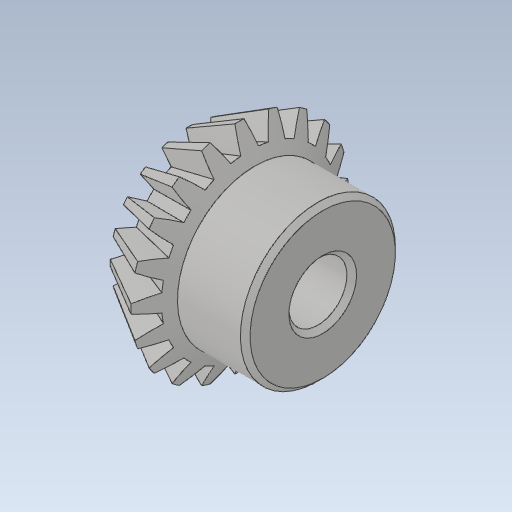
# Autodesk Inventor part: PB1-2040_On
Saved by Autodesk Inventor 2024 (Build 280153000, 153)
## iProperties
Created: 2023-09-03
Part Number: PB1-2040_On
Material: Generic
Catalog Web Link: www.cadenas.de
Description: Plastic Bevel Gears (PB)-L-
Vendor: KHK
Document SubType Name: Modeling
Designer: psAdmin
Manufacturer: KHK
Mass: 2.44535 g
Surface Area: 17.1711 cm^2
Volume: 2.44535 cm^3
Density: 1 g/cm^3
Appearance: PSOLRGB-175-175-175
Category: PARTsolutions
Company: KHK
PSOL_IDENT_0: {$CADENAS_DATA/23d-libs/khk/bevel_gears/pb_l.prj},185 {VTYP=3D},{NB=PB1-2040_On},{LINA=PB1-2040},{NN=
PSOL_IDENT_1: Plastic Bevel Gears (PB)-L},{DATE=06.10.2022 23:14:38},{GEOMDATE=20.03.2019 11:23:50},{VERSION=},{LI
PSOL_IDENT_2: NEID=110},{WBVAR=TOOTH},{WBNUMERIC=}  {NB=PB1-2040_On},{LINA=PB1-2040},{KT=DUMMY},{CN=PB1-2040},{M=1
PSOL_IDENT_3: .0},{Z=20},{A=6},{B=16},{C=20.0},{D=22.41},{E=28},{F=13.78},{G=8.60},{H=7.00},{I=12.0},{J=6},{K=9.17
PSOL_IDENT_4: },{L=30.48},{S=B3},{PN=PB1-4020},{WMF=B3010.WMF},{X=0.5},{Y=0.5},{R=0.0},{H1=0.00},{VERS=5},{TOOTH=O
PSOL_IDENT_5: n},{ANGLE=27.000}
NB: PB1-2040_On
NN: Plastic Bevel Gears (PB)-L
NBSYN: $CN._$TOOTH.
LINA: PB1-2040
CATALOG: KHK
CN: PB1-2040
M: 1
Z: 20
A: 6
B: 16
C: 20
D: 22.41
E: 28
F: 13.78
G: 8.6
H: 7
I: 12
J: 6
K: 9.17
L: 30.48
S: B3
PN: PB1-4020
WMF: B3010.WMF
X: 0.5
Y: 0.5
R: 0
H1: 0
VERS: 5
TOOTH: On
ANGLE: 27
SUPPLIER: KHK
ARTICLENO: PB1-2040_On
BOMINFO: PB1-2040
CREATOR: CADENAS GmbH
Title: PB1-2040
Author: Cadenas PARTsolutions
Autodesk Inventor part; units mm, degrees
sketch "Sketch_4" plane through (21, 0, 0) normal (1, 0, 0) x (0, 0, -1)
  arc A0 (-0.3956, 12.5887) -> (-0.9758, 8.8384) centre (21.3814, 7.2999) ccw
  arc A1 (-0.9758, 8.8384) -> (-1.8032, 8.7074) centre (0, 0) ccw
  arc A2 (-1.8032, 8.7074) -> (-3.5139, 12.0948) centre (-22.5907, 0.3354) ccw
  arc A3 (-3.5139, 12.0948) -> (-4.2664, 11.8503) centre (0, 0) ccw
  arc A4 (-4.2664, 11.8503) -> (-3.6592, 8.1043) centre (18.0791, 13.5498) ccw
  arc A5 (-3.6592, 8.1043) -> (-4.4057, 7.724) centre (0, 0) ccw
  arc A6 (-4.4057, 7.724) -> (-7.0794, 10.417) centre (-21.5886, -6.6619) ccw
  arc A7 (-7.0794, 10.417) -> (-7.7195, 9.9519) centre (0, 0) ccw
  arc A8 (-7.7195, 9.9519) -> (-5.9845, 6.5769) centre (13.0071, 18.4734) ccw
  arc A9 (-5.9845, 6.5769) -> (-6.5769, 5.9845) centre (0, 0) ccw
  arc A10 (-6.5769, 5.9845) -> (-9.9519, 7.7195) centre (-18.4734, -13.0071) ccw
  arc A11 (-9.9519, 7.7195) -> (-10.417, 7.0794) centre (0, 0) ccw
  arc A12 (-10.417, 7.0794) -> (-7.724, 4.4057) centre (6.6619, 21.5886) ccw
  arc A13 (-7.724, 4.4057) -> (-8.1043, 3.6592) centre (0, 0) ccw
  arc A14 (-8.1043, 3.6592) -> (-11.8503, 4.2664) centre (-13.5498, -18.0791) ccw
  arc A15 (-11.8503, 4.2664) -> (-12.0948, 3.5139) centre (0, 0) ccw
  arc A16 (-12.0948, 3.5139) -> (-8.7074, 1.8032) centre (-0.3354, 22.5907) ccw
  arc A17 (-8.7074, 1.8032) -> (-8.8384, 0.9758) centre (0, 0) ccw
  arc A18 (-8.8384, 0.9758) -> (-12.5887, 0.3956) centre (-7.2999, -21.3814) ccw
  arc A19 (-12.5887, 0.3956) -> (-12.5887, -0.3956) centre (0, 0) ccw
  arc A20 (-12.5887, -0.3956) -> (-8.8384, -0.9758) centre (-7.2999, 21.3814) ccw
  arc A21 (-8.8384, -0.9758) -> (-8.7074, -1.8032) centre (0, 0) ccw
  arc A22 (-8.7074, -1.8032) -> (-12.0948, -3.5139) centre (-0.3354, -22.5907) ccw
  arc A23 (-12.0948, -3.5139) -> (-11.8503, -4.2664) centre (0, 0) ccw
  arc A24 (-11.8503, -4.2664) -> (-8.1043, -3.6592) centre (-13.5498, 18.0791) ccw
  arc A25 (-8.1043, -3.6592) -> (-7.724, -4.4057) centre (0, 0) ccw
  arc A26 (-7.724, -4.4057) -> (-10.417, -7.0794) centre (6.6619, -21.5886) ccw
  arc A27 (-10.417, -7.0794) -> (-9.9519, -7.7195) centre (0, 0) ccw
  arc A28 (-9.9519, -7.7195) -> (-6.5769, -5.9845) centre (-18.4734, 13.0071) ccw
  arc A29 (-6.5769, -5.9845) -> (-5.9845, -6.5769) centre (0, 0) ccw
  arc A30 (-5.9845, -6.5769) -> (-7.7195, -9.9519) centre (13.0071, -18.4734) ccw
  arc A31 (-7.7195, -9.9519) -> (-7.0794, -10.417) centre (0, 0) ccw
  arc A32 (-7.0794, -10.417) -> (-4.4057, -7.724) centre (-21.5886, 6.6619) ccw
  arc A33 (-4.4057, -7.724) -> (-3.6592, -8.1043) centre (0, 0) ccw
  arc A34 (-3.6592, -8.1043) -> (-4.2664, -11.8503) centre (18.0791, -13.5498) ccw
  arc A35 (-4.2664, -11.8503) -> (-3.5139, -12.0948) centre (0, 0) ccw
  arc A36 (-3.5139, -12.0948) -> (-1.8032, -8.7074) centre (-22.5907, -0.3354) ccw
  arc A37 (-1.8032, -8.7074) -> (-0.9758, -8.8384) centre (0, 0) ccw
  arc A38 (-0.9758, -8.8384) -> (-0.3956, -12.5887) centre (21.3814, -7.2999) ccw
  arc A39 (-0.3956, -12.5887) -> (0.3956, -12.5887) centre (0, 0) ccw
  arc A40 (0.3956, -12.5887) -> (0.9758, -8.8384) centre (-21.3814, -7.2999) ccw
  arc A41 (0.9758, -8.8384) -> (1.8032, -8.7074) centre (0, 0) ccw
  arc A42 (1.8032, -8.7074) -> (3.5139, -12.0948) centre (22.5907, -0.3354) ccw
  arc A43 (3.5139, -12.0948) -> (4.2664, -11.8503) centre (0, 0) ccw
  arc A44 (4.2664, -11.8503) -> (3.6592, -8.1043) centre (-18.0791, -13.5498) ccw
  arc A45 (3.6592, -8.1043) -> (4.4057, -7.724) centre (0, 0) ccw
  arc A46 (4.4057, -7.724) -> (7.0794, -10.417) centre (21.5886, 6.6619) ccw
  arc A47 (7.0794, -10.417) -> (7.7195, -9.9519) centre (0, 0) ccw
  arc A48 (7.7195, -9.9519) -> (5.9845, -6.5769) centre (-13.0071, -18.4734) ccw
  arc A49 (5.9845, -6.5769) -> (6.5769, -5.9845) centre (0, 0) ccw
  arc A50 (6.5769, -5.9845) -> (9.9519, -7.7195) centre (18.4734, 13.0071) ccw
  arc A51 (9.9519, -7.7195) -> (10.417, -7.0794) centre (0, 0) ccw
  arc A52 (10.417, -7.0794) -> (7.724, -4.4057) centre (-6.6619, -21.5886) ccw
  arc A53 (7.724, -4.4057) -> (8.1043, -3.6592) centre (0, 0) ccw
  arc A54 (8.1043, -3.6592) -> (11.8503, -4.2664) centre (13.5498, 18.0791) ccw
  arc A55 (11.8503, -4.2664) -> (12.0948, -3.5139) centre (0, 0) ccw
  arc A56 (12.0948, -3.5139) -> (8.7074, -1.8032) centre (0.3354, -22.5907) ccw
  arc A57 (8.7074, -1.8032) -> (8.8384, -0.9758) centre (0, 0) ccw
  arc A58 (8.8384, -0.9758) -> (12.5887, -0.3956) centre (7.2999, 21.3814) ccw
  arc A59 (12.5887, -0.3956) -> (12.5887, 0.3956) centre (0, 0) ccw
  arc A60 (12.5887, 0.3956) -> (8.8384, 0.9758) centre (7.2999, -21.3814) ccw
  arc A61 (8.8384, 0.9758) -> (8.7074, 1.8032) centre (0, 0) ccw
  arc A62 (8.7074, 1.8032) -> (12.0948, 3.5139) centre (0.3354, 22.5907) ccw
  arc A63 (12.0948, 3.5139) -> (11.8503, 4.2664) centre (0, 0) ccw
  arc A64 (11.8503, 4.2664) -> (8.1043, 3.6592) centre (13.5498, -18.0791) ccw
  arc A65 (8.1043, 3.6592) -> (7.724, 4.4057) centre (0, 0) ccw
  arc A66 (7.724, 4.4057) -> (10.417, 7.0794) centre (-6.6619, 21.5886) ccw
  arc A67 (10.417, 7.0794) -> (9.9519, 7.7195) centre (0, 0) ccw
  arc A68 (9.9519, 7.7195) -> (6.5769, 5.9845) centre (18.4734, -13.0071) ccw
  arc A69 (6.5769, 5.9845) -> (5.9845, 6.5769) centre (0, 0) ccw
  arc A70 (5.9845, 6.5769) -> (7.7195, 9.9519) centre (-13.0071, 18.4734) ccw
  arc A71 (7.7195, 9.9519) -> (7.0794, 10.417) centre (0, 0) ccw
  arc A72 (7.0794, 10.417) -> (4.4057, 7.724) centre (21.5886, -6.6619) ccw
  arc A73 (4.4057, 7.724) -> (3.6592, 8.1043) centre (0, 0) ccw
  arc A74 (3.6592, 8.1043) -> (4.2664, 11.8503) centre (-18.0791, 13.5498) ccw
  arc A75 (4.2664, 11.8503) -> (3.5139, 12.0948) centre (0, 0) ccw
  arc A76 (3.5139, 12.0948) -> (1.8032, 8.7074) centre (22.5907, 0.3354) ccw
  arc A77 (1.8032, 8.7074) -> (0.9758, 8.8384) centre (0, 0) ccw
  arc A78 (0.9758, 8.8384) -> (0.3956, 12.5887) centre (-21.3814, 7.2999) ccw
  arc A79 (0.3956, 12.5887) -> (-0.3956, 12.5887) centre (0, 0) ccw
  constraints: 160 point on circle, 80 centre point
sketch "Sketch_5" plane through (14.22, 0, 0) normal (1, 0, 0) x (0, 0, -1)
  arc A0 (-0.2219, 8.8257) -> (-0.538, 5.6918) centre (21.8617, 5.0148) ccw
  arc A1 (-0.538, 5.6918) -> (-1.2472, 5.5795) centre (0, 0) ccw
  arc A2 (-1.2472, 5.5795) -> (-2.5163, 8.4623) centre (-22.3414, -1.9863) ccw
  arc A3 (-2.5163, 8.4623) -> (-2.9383, 8.3252) centre (0, 0) ccw
  arc A4 (-2.9383, 8.3252) -> (-2.2706, 5.247) centre (19.2421, 11.525) ccw
  arc A5 (-2.2706, 5.247) -> (-2.9103, 4.921) centre (0, 0) ccw
  arc A6 (-2.9103, 4.921) -> (-5.0081, 7.2705) centre (-20.6342, -8.7929) ccw
  arc A7 (-5.0081, 7.2705) -> (-5.3671, 7.0097) centre (0, 0) ccw
  arc A8 (-5.3671, 7.0097) -> (-3.7808, 4.2885) centre (14.7389, 16.9071) ccw
  arc A9 (-3.7808, 4.2885) -> (-4.2885, 3.7808) centre (0, 0) ccw
  arc A10 (-4.2885, 3.7808) -> (-7.0097, 5.3671) centre (-16.9071, -14.7389) ccw
  arc A11 (-7.0097, 5.3671) -> (-7.2705, 5.0081) centre (0, 0) ccw
  arc A12 (-7.2705, 5.0081) -> (-4.921, 2.9103) centre (8.7929, 20.6342) ccw
  arc A13 (-4.921, 2.9103) -> (-5.247, 2.2706) centre (0, 0) ccw
  arc A14 (-5.247, 2.2706) -> (-8.3252, 2.9383) centre (-11.525, -19.2421) ccw
  arc A15 (-8.3252, 2.9383) -> (-8.4623, 2.5163) centre (0, 0) ccw
  arc A16 (-8.4623, 2.5163) -> (-5.5795, 1.2472) centre (1.9863, 22.3414) ccw
  arc A17 (-5.5795, 1.2472) -> (-5.6918, 0.538) centre (0, 0) ccw
  arc A18 (-5.6918, 0.538) -> (-8.8257, 0.2219) centre (-5.0148, -21.8617) ccw
  arc A19 (-8.8257, 0.2219) -> (-8.8257, -0.2219) centre (0, 0) ccw
  arc A20 (-8.8257, -0.2219) -> (-5.6918, -0.538) centre (-5.0148, 21.8617) ccw
  arc A21 (-5.6918, -0.538) -> (-5.5795, -1.2472) centre (0, 0) ccw
  arc A22 (-5.5795, -1.2472) -> (-8.4623, -2.5163) centre (1.9863, -22.3414) ccw
  arc A23 (-8.4623, -2.5163) -> (-8.3252, -2.9383) centre (0, 0) ccw
  arc A24 (-8.3252, -2.9383) -> (-5.247, -2.2706) centre (-11.525, 19.2421) ccw
  arc A25 (-5.247, -2.2706) -> (-4.921, -2.9103) centre (0, 0) ccw
  arc A26 (-4.921, -2.9103) -> (-7.2705, -5.0081) centre (8.7929, -20.6342) ccw
  arc A27 (-7.2705, -5.0081) -> (-7.0097, -5.3671) centre (0, 0) ccw
  arc A28 (-7.0097, -5.3671) -> (-4.2885, -3.7808) centre (-16.9071, 14.7389) ccw
  arc A29 (-4.2885, -3.7808) -> (-3.7808, -4.2885) centre (0, 0) ccw
  arc A30 (-3.7808, -4.2885) -> (-5.3671, -7.0097) centre (14.7389, -16.9071) ccw
  arc A31 (-5.3671, -7.0097) -> (-5.0081, -7.2705) centre (0, 0) ccw
  arc A32 (-5.0081, -7.2705) -> (-2.9103, -4.921) centre (-20.6342, 8.7929) ccw
  arc A33 (-2.9103, -4.921) -> (-2.2706, -5.247) centre (0, 0) ccw
  arc A34 (-2.2706, -5.247) -> (-2.9383, -8.3252) centre (19.2421, -11.525) ccw
  arc A35 (-2.9383, -8.3252) -> (-2.5163, -8.4623) centre (0, 0) ccw
  arc A36 (-2.5163, -8.4623) -> (-1.2472, -5.5795) centre (-22.3414, 1.9863) ccw
  arc A37 (-1.2472, -5.5795) -> (-0.538, -5.6918) centre (0, 0) ccw
  arc A38 (-0.538, -5.6918) -> (-0.2219, -8.8257) centre (21.8617, -5.0148) ccw
  arc A39 (-0.2219, -8.8257) -> (0.2219, -8.8257) centre (0, 0) ccw
  arc A40 (0.2219, -8.8257) -> (0.538, -5.6918) centre (-21.8617, -5.0148) ccw
  arc A41 (0.538, -5.6918) -> (1.2472, -5.5795) centre (0, 0) ccw
  arc A42 (1.2472, -5.5795) -> (2.5163, -8.4623) centre (22.3414, 1.9863) ccw
  arc A43 (2.5163, -8.4623) -> (2.9383, -8.3252) centre (0, 0) ccw
  arc A44 (2.9383, -8.3252) -> (2.2706, -5.247) centre (-19.2421, -11.525) ccw
  arc A45 (2.2706, -5.247) -> (2.9103, -4.921) centre (0, 0) ccw
  arc A46 (2.9103, -4.921) -> (5.0081, -7.2705) centre (20.6342, 8.7929) ccw
  arc A47 (5.0081, -7.2705) -> (5.3671, -7.0097) centre (0, 0) ccw
  arc A48 (5.3671, -7.0097) -> (3.7808, -4.2885) centre (-14.7389, -16.9071) ccw
  arc A49 (3.7808, -4.2885) -> (4.2885, -3.7808) centre (0, 0) ccw
  arc A50 (4.2885, -3.7808) -> (7.0097, -5.3671) centre (16.9071, 14.7389) ccw
  arc A51 (7.0097, -5.3671) -> (7.2705, -5.0081) centre (0, 0) ccw
  arc A52 (7.2705, -5.0081) -> (4.921, -2.9103) centre (-8.7929, -20.6342) ccw
  arc A53 (4.921, -2.9103) -> (5.247, -2.2706) centre (0, 0) ccw
  arc A54 (5.247, -2.2706) -> (8.3252, -2.9383) centre (11.525, 19.2421) ccw
  arc A55 (8.3252, -2.9383) -> (8.4623, -2.5163) centre (0, 0) ccw
  arc A56 (8.4623, -2.5163) -> (5.5795, -1.2472) centre (-1.9863, -22.3414) ccw
  arc A57 (5.5795, -1.2472) -> (5.6918, -0.538) centre (0, 0) ccw
  arc A58 (5.6918, -0.538) -> (8.8257, -0.2219) centre (5.0148, 21.8617) ccw
  arc A59 (8.8257, -0.2219) -> (8.8257, 0.2219) centre (0, 0) ccw
  arc A60 (8.8257, 0.2219) -> (5.6918, 0.538) centre (5.0148, -21.8617) ccw
  arc A61 (5.6918, 0.538) -> (5.5795, 1.2472) centre (0, 0) ccw
  arc A62 (5.5795, 1.2472) -> (8.4623, 2.5163) centre (-1.9863, 22.3414) ccw
  arc A63 (8.4623, 2.5163) -> (8.3252, 2.9383) centre (0, 0) ccw
  arc A64 (8.3252, 2.9383) -> (5.247, 2.2706) centre (11.525, -19.2421) ccw
  arc A65 (5.247, 2.2706) -> (4.921, 2.9103) centre (0, 0) ccw
  arc A66 (4.921, 2.9103) -> (7.2705, 5.0081) centre (-8.7929, 20.6342) ccw
  arc A67 (7.2705, 5.0081) -> (7.0097, 5.3671) centre (0, 0) ccw
  arc A68 (7.0097, 5.3671) -> (4.2885, 3.7808) centre (16.9071, -14.7389) ccw
  arc A69 (4.2885, 3.7808) -> (3.7808, 4.2885) centre (0, 0) ccw
  arc A70 (3.7808, 4.2885) -> (5.3671, 7.0097) centre (-14.7389, 16.9071) ccw
  arc A71 (5.3671, 7.0097) -> (5.0081, 7.2705) centre (0, 0) ccw
  arc A72 (5.0081, 7.2705) -> (2.9103, 4.921) centre (20.6342, -8.7929) ccw
  arc A73 (2.9103, 4.921) -> (2.2706, 5.247) centre (0, 0) ccw
  arc A74 (2.2706, 5.247) -> (2.9383, 8.3252) centre (-19.2421, 11.525) ccw
  arc A75 (2.9383, 8.3252) -> (2.5163, 8.4623) centre (0, 0) ccw
  arc A76 (2.5163, 8.4623) -> (1.2472, 5.5795) centre (22.3414, -1.9863) ccw
  arc A77 (1.2472, 5.5795) -> (0.538, 5.6918) centre (0, 0) ccw
  arc A78 (0.538, 5.6918) -> (0.2219, 8.8257) centre (-21.8617, 5.0148) ccw
  arc A79 (0.2219, 8.8257) -> (-0.2219, 8.8257) centre (0, 0) ccw
  constraints: 160 point on circle, 80 centre point
loft "Loft1" add profiles "Sketch_5", "Sketch_4"
sketch "Sketch_6" plane through (0, 0, 0) normal (0, 0, 1) x (1, 0, 0)
  line L0 (28, 0) -> (14.22, 0)
  line L1 (16, 0) -> (16, 4.585)
  line L2 (16, 4.585) -> (14.9436, 6.7044)
  line L3 (14.9436, 6.7044) -> (20.4503, 9.1011)
  line L4 (20.4503, 9.1011) -> (21, 8)
  line L5 (21, 8) -> (27.5, 8)
  line L6 (27.5, 8) -> (28, 7.5)
  line L7 (28, 7.5) -> (28, 0)
  line L8 (28, 0) -> (16, 0)
  constraints: 18 end point
revolve "Revolution1" add sketch "Sketch_6" angle 360 about axis through (28, 0, 0) along (1, 0, 0)
sketch "Sketch_7" plane through (0, 0, 0) normal (0, 0, 1) x (1, 0, 0)
  line L0 (28, 0) -> (14.22, 0)
  line L1 (0, 0) -> (0, 22.41)
  line L2 (0, 22.41) -> (21, 22.41)
  line L3 (21, 22.41) -> (21, 8)
  line L4 (21, 8) -> (19.4, 11.205)
  line L5 (19.4, 11.205) -> (14.22, 8.1562)
  line L6 (14.22, 8.1562) -> (16, 4.585)
  line L7 (16, 4.585) -> (16, 3.5)
  line L8 (16, 3.5) -> (16.5, 3)
  line L9 (16.5, 3) -> (27.5, 3)
  line L10 (27.5, 3) -> (28, 3.5)
  line L11 (28, 3.5) -> (28, 0)
  line L12 (28, 0) -> (0, 0)
  constraints: 26 end point
revolve "Revolution2" cut sketch "Sketch_7" angle 360 about axis through (28, 0, 0) along (1, 0, 0)
ref_plane "IP2_XY" through (0, 0, 0) normal (1, 0, 0) x (0, 0, -1)
ref_plane "IP2_YZ" through (0, 0, 0) normal (0, 0, -1) x (0, 1, 0)
ref_plane "IP2_ZX" through (0, 0, 0) normal (0, 1, 0) x (1, 0, 0)
ref_plane "l_XY" through (0, 0, 0) normal (0, 1, 0) x (1, 0, 0)
ref_plane "l_YZ" through (0, 0, 0) normal (1, 0, 0) x (0, 0, -1)
ref_plane "l_ZX" through (0, 0, 0) normal (0, 0, -1) x (0, 1, 0)
body "Solid1"
